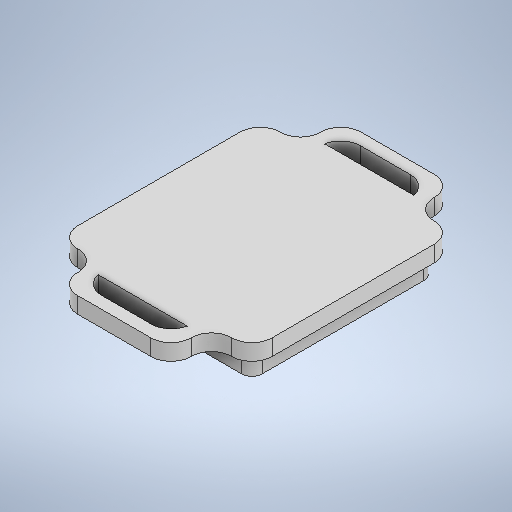
# Autodesk Inventor part: PCB_Mount
Saved by Autodesk Inventor 2025.2 (Build 292293000, 293)
## iProperties
Created: 2024-11-12
Part Number: PCB_Mount
Material: Generic
Document SubType Name: Modeling
Designer: matss
Density: 1 g/cm^3
Appearance: Default
Author: matss
Autodesk Inventor part; units mm, degrees
ref_plane "YZ Plane" through (0, 0, 0) normal (1, 0, 0) x (0, 1, 0)
ref_plane "XZ Plane" through (0, 0, 0) normal (0, 1, 0) x (-1, 0, 0)
ref_plane "XY Plane" through (0, 0, 0) normal (0, 0, 1) x (1, 0, 0)
sketch "Sketch1" plane through (0, 0, 0) normal (0, 1, 0) x (-1, 0, 0)
  line L0 (0, 14.23) -> (0, -14.23) construction
  circle A0 centre (0, 14.23) radius 1
  circle A1 centre (0, -14.23) radius 1
  line L1 (10, 25) -> (-38, 25)
  line L2 (-38, 25) -> (-38, -25)
  line L3 (-38, -25) -> (10, -25)
  line L4 (10, -25) -> (10, 25)
  point P0 (0, 0)
  point P1 (0, 0)
  point P2 (10, 0)
  dimension "d0" = 28.46
  dimension "d1" = 2
  dimension "d2" = 2
  dimension "d3" = 50
  dimension "d4" = 48
  dimension "d5" = 10
  constraints: 10 end point, 3 coincident, 2 centre point, 2 midpoint, 2 parallel, 1 horizontal, 1 horizontal alignment, 1 perpendicular
  measures "d0" distance of L0.start L0.end
  measures "d1" diameter of A0
  measures "d2" diameter of A1
  measures "d3" distance of L3.end L1.start
  measures "d4" distance between parallel lines of L2 L4
  measures "d5" distance between parallel lines of L0 L4
extrude "Extrusion1" add sketch "Sketch1" along normal blind 4 contours A0 | A1 | L4 L3 L2 L1
extrude "Extrusion2" add sketch "Sketch1" against normal blind 5 contours A0 | A1
sketch "Sketch2" plane through (0, 0, 0) normal (0, -1, 0) x (1, 0, 0)
  line L0 (24, -10) -> (29, -10)
  line L1 (29, -10) -> (29, -5)
  line L2 (29, -5) -> (24, -5)
  line L3 (24, -5) -> (24, -10)
  line L4 (38, 25) -> (38, -25) projected
  line L5 (38, -25) -> (-10, -25) projected
  point P0 (0, 0)
  dimension "d10" = 5
  dimension "d11" = 5
  dimension "d12" = 9
  dimension "d13" = 15
  constraints: 8 end point, 2 parallel, 1 horizontal, 1 perpendicular
  measures "d10" distance of L2.end L0.start
  measures "d11" distance of L0.start L0.end
  measures "d12" distance between parallel lines of L4 L1
  measures "d13" distance between parallel lines of L5 L0
extrude "Extrusion3" add sketch "Sketch2" along normal blind 2.5
sketch "Sketch3" plane through (0, 0, 0) normal (0, -1, 0) x (1, 0, 0)
  line L0 (-1, -5) -> (1, -5)
  line L1 (1, -5) -> (1, 5)
  line L2 (1, 5) -> (-1, 5)
  line L3 (-1, 5) -> (-1, -5)
  circle A0 centre (0, 14.23) radius 1 projected
  circle A1 centre (0, -14.23) radius 1 projected
  circle A2 centre (0, 14.23) radius 1 projected
  circle A3 centre (0, -14.23) radius 1 projected
  point P0 (0, 0)
  point P1 (0, -5)
  point P2 (-1, 0)
  dimension "d16" = 2
  dimension "d17" = 10
  constraints: 8 end point, 2 midpoint, 2 parallel, 1 horizontal, 1 horizontal alignment, 1 perpendicular, 1 vertical alignment
  measures "d16" distance of L1.end L2.end
  measures "d17" distance of L2.end L0.start
extrude "Extrusion4" add sketch "Sketch3" along normal blind 2.5 contours L3 L2 L1 L0
fillet "Fillet1" radius 0.5 8 edges at (-1, -1.25, -5) (1, -1.25, -5) (1, -1.25, 5) (-1, -1.25, 5) (24, -1.25, -10) (24, -1.25, -5) (29, -1.25, -10) (29, -1.25, -5)
chamfer "Chamfer2" distance 0.5 angle 45 2 edges at (1, 0, -14.23) (1, 0, 14.23)
fillet "Fillet2" radius 5 4 edges at (38, 2, -25) (38, 2, 25) (-10, 2, 25) (-10, 2, -25)
sketch "Sketch6" plane through (0, 4, 0) normal (0, 1, 0) x (1, 0, 0)
  line L0 (-5, -25) -> (33, -25) projected
  line L1 (-10, 20) -> (-10, -20) projected
  line L2 (38, -20) -> (38, 20) projected
  line L3 (33, 25) -> (-5, 25) projected
  line L4 (-10, 0) -> (38, 0) construction
  line L5 (3, -32) -> (25, -32)
  line L6 (25, -32) -> (25, -28)
  line L7 (25, -28) -> (3, -28)
  line L8 (3, -28) -> (3, -32)
  line L9 (0, -35) -> (28, -35)
  line L10 (28, -35) -> (28, -25)
  line L11 (28, -25) -> (0, -25)
  line L12 (0, -25) -> (0, -35)
  line L13 (0, -30) -> (3, -30) construction
  line L14 (14, -35) -> (14, -32) construction
  line L15 (3, 32) -> (25, 32)
  line L16 (25, 32) -> (25, 28)
  line L17 (25, 28) -> (3, 28)
  line L18 (3, 28) -> (3, 32)
  line L19 (0, 35) -> (28, 35)
  line L20 (28, 35) -> (28, 25)
  line L21 (28, 25) -> (0, 25)
  line L22 (0, 25) -> (0, 35)
  point P0 (0, 0)
  point P1 (14, -28)
  point P2 (14, -25)
  point P3 (14, -25)
  point P4 (3, 30)
  dimension "d32" = 5
  dimension "d33" = 3
  dimension "d34" = 4
  constraints: 38 end point, 9 midpoint, 9 symmetric about line, 4 parallel, 3 horizontal, 3 perpendicular, 3 vertical alignment, 1 horizontal alignment, 1 point on line, 1 vertical
  measures "d32" distance of L11.end L0.start
  measures "d33" distance of L13.start L13.end
  measures "d34" distance between parallel lines of L5 L7
extrude "Extrusion6" add sketch "Sketch6" against normal up to surface (4 mm away)
fillet "Fillet3" radius 5 12 edges at (28, 2, -25) (28, 2, 25) (28, 2, 35) (0, 2, 35) (0, 2, 25) (3, 2, 32) (25, 2, 32) (0, 2, -25) (0, 2, -35) (28, 2, -35) (3, 2, -32) (25, 2, -32)
sketch "Sketch7" plane through (0, 0, 0) normal (0, -1, 0) x (1, 0, 0)
  arc A0 (-10, -20) -> (-5, -25) centre (-5, -20) ccw projected
  line L0 (-10, -20) -> (-10, 20) projected
  arc A1 (-5, 25) -> (-10, 20) centre (-5, 20) ccw projected
  arc A2 (38, 20) -> (33, 25) centre (33, 20) ccw projected
  line L1 (38, 20) -> (38, -20) projected
  arc A3 (33, -25) -> (38, -20) centre (33, -20) ccw projected
  arc A4 (33, -25) -> (28, -30) centre (33, -30) ccw projected
  line L2 (-5, -25) -> (33, -25)
  arc A5 (-5, 25) -> (-10, 20) centre (-5, 20) ccw projected
  line L3 (-5, 25) -> (33, 25)
  line L4 (-7.5, 20) -> (-7.5, -20)
  arc A6 (-7.5, -20) -> (-5, -22.5) centre (-5, -20) ccw
  line L5 (-5, -22.5) -> (33, -22.5)
  arc A7 (33, -22.5) -> (35.5, -20) centre (33, -20) ccw
  line L6 (35.5, -20) -> (35.5, 20)
  arc A8 (35.5, 20) -> (33, 22.5) centre (33, 20) ccw
  line L7 (33, 22.5) -> (-5, 22.5)
  arc A9 (-5, 22.5) -> (-7.5, 20) centre (-5, 20) ccw
  line L8 (-5.5, -20) -> (-5.5, 20)
  arc A10 (-5, 20.5) -> (-5.5, 20) centre (-5, 20) ccw
  line L9 (-5, 20.5) -> (33, 20.5)
  arc A11 (33.5, 20) -> (33, 20.5) centre (33, 20) ccw
  line L10 (33.5, 20) -> (33.5, -20)
  arc A12 (33, -20.5) -> (33.5, -20) centre (33, -20) ccw
  line L11 (33, -20.5) -> (-5, -20.5)
  arc A13 (-5.5, -20) -> (-5, -20.5) centre (-5, -20) ccw
  point P0 (0, 0)
  dimension "d38" = 2.5
  dimension "d39" = 2
  constraints: 20 end point, 16 point on circle, 8 centre point, 4 tangent, 2 horizontal, 1 coincident, 13 other
  measures "d38" distance between parallel lines of L0 L4
  measures "d39" distance between parallel lines of L4 L8
extrude "Extrusion7" add sketch "Sketch7" along normal blind 5 contours A9 L7 A8 L6 A7 L5 A6 L4
body "Solid1"
